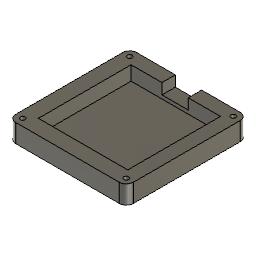
Abhay's+Macropad+Bottom (Autodesk Fusion 360 design; units mm, degrees)
part number: 2026-01-28-15-56-50-540
Autodesk Fusion 360 part; units mm, degrees
sketch "Sketch1" plane through (0, 0, 0) normal (0, 0, 1) x (1, 0, 0)
  line L0 (55, 35) -> (117.913, 35)
  line L1 (117.913, 35) -> (117.913, -30.294)
  line L2 (117.913, -30.294) -> (55, -30.294)
  line L3 (55, -30.294) -> (55, 35)
  line L4 (44.5, -40.794) -> (127.413, -40.794)
  line L5 (127.413, -40.794) -> (127.413, 44.5)
  line L6 (127.413, 44.5) -> (44.5, 44.5)
  line L7 (44.5, 44.5) -> (44.5, -40.794)
  circle A0 centre (49.5, -35.794) radius 1.7
  circle A1 centre (49.5, 39.5) radius 1.7
  circle A2 centre (122.413, 39.5) radius 1.7
  circle A3 centre (122.413, -35.794) radius 1.7
  circle A4 centre (49.5, -35.794) radius 3
  circle A5 centre (49.5, 39.5) radius 3
  circle A6 centre (122.413, 39.5) radius 3
  circle A7 centre (122.413, -35.794) radius 3
  dimension "d1" = 62.913
  dimension "d2" = 65.294
  dimension "d3" = 82.913
  dimension "d4" = 85.294
  dimension "d5" = 9.5
  dimension "d6" = 9.5
  dimension "d7" = 3.4
  dimension "d8" = 3.4
  dimension "d9" = 3.4
  dimension "d10" = 3.4
  dimension "d11" = 5
  dimension "d12" = 5
  dimension "d13" = 5
  dimension "d14" = 5
  dimension "d15" = 5
  dimension "d16" = 5
  dimension "d17" = 5
  dimension "d18" = 5
  dimension "d19" = 6
  dimension "d20" = 6
  dimension "d21" = 6
  dimension "d22" = 6
  constraint horizontal L0
  constraint vertical L1
  constraint horizontal L2
  constraint vertical L3
  constraint horizontal L4
  constraint vertical L5
  constraint horizontal L6
  constraint vertical L7
  constraint concentric A0 A4
  constraint concentric A1 A5
  constraint concentric A2 A6
  constraint concentric A3 A7
  measures "d1" distance of L0.start L0.end
  measures "d2" distance of L0.start L2.end
  measures "d3" distance of L4.start L4.end
  measures "d4" distance of L4.start L6.end
  measures "d5" distance of L0 L6
  measures "d6" distance of L1 L5
  measures "d7" diameter of A0
  measures "d8" diameter of A1
  measures "d9" diameter of A2
  measures "d10" diameter of A3
  measures "d11" distance of L4 A3.centre
  measures "d12" distance of L5 A3.centre
  measures "d13" distance of L6 A2.centre
  measures "d14" distance of L5 A2.centre
  measures "d15" distance of L6 A1.centre
  measures "d16" distance of L7 A1.centre
  measures "d17" distance of L4 A0.centre
  measures "d18" distance of L7 A0.centre
  measures "d19" diameter of A4
  measures "d20" diameter of A5
  measures "d21" diameter of A6
  measures "d22" diameter of A7
extrude "Extrude1" add sketch "Sketch1" along normal blind 9.9 from surface at 3.1 contours A4 | A5 | A6 | A7 makes body 1 at (123.2255, -32.9061, 9.7) makes body 2 at (123.2255, 42.3879, 9.7) makes body 3 at (46.5037, -35.9435, 9.7) makes body 4 at (46.5037, 39.3505, 9.7)
extrude "Extrude2" add sketch "Sketch1" along normal blind 13 contours L4 L5 L6 L7 bodies 1 2 3 4
extrude "Extrude3" add sketch "Sketch1" along normal blind 3 contours L0 L1 L2 L3 bodies 1
sketch "Sketch2" plane through (0, 0, 13) normal (0, 0, 1) x (-1, 0, 0)
  circle A0 centre (-122.413, 35.794) radius 1.7
  circle A1 centre (-49.5, -39.5) radius 1.7
  line L0 (-117.913, 30.294) -> (-55, 30.294)
  line L1 (-55, 30.294) -> (-55, -35)
  line L2 (-55, -35) -> (-117.913, -35)
  line L3 (-117.913, -35) -> (-117.913, 30.294)
  line L4 (-44.5, -44.5) -> (-44.5, 40.794)
  line L5 (-44.5, 40.794) -> (-127.413, 40.794)
  line L6 (-127.413, 40.794) -> (-127.413, -44.5)
  line L7 (-127.413, -44.5) -> (-44.5, -44.5)
  circle A2 centre (-122.413, -39.5) radius 1.7
  circle A3 centre (-49.5, 35.794) radius 1.7
  line L8 (-76.7065, -44.5) -> (-95.2065, -44.5)
  line L9 (-95.2065, -44.5) -> (-95.2065, -35)
  line L10 (-95.2065, -35) -> (-76.7065, -35)
  line L11 (-76.7065, -35) -> (-76.7065, -44.5)
  line L12 (-44.5, -44.5) -> (-44.5, 40.794)
  dimension "d30" = 18.5
  dimension "d31" = 32.2065
  constraint horizontal L8
  constraint vertical L9
  constraint horizontal L10
  constraint vertical L11
  constraint coincident L7 L8.start
  measures "d30" distance of L8.start L8.end
  measures "d31" distance of L11 L12
extrude "Extrude4" cut sketch "Sketch2" against normal blind 7.5 contours L2 L7 L8 L9 L10 L11 bodies 1
fillet "Fillet1" radius 5 4 edges at (44.5, 44.5, 6.5) (44.5, -40.794, 6.5) (127.413, 44.5, 6.5) (127.413, -40.794, 6.5) on bodies 1
sketch "Sketch3" plane through (0, 0, 13) normal (0, 0, 1) x (-1, 0, 0)
  circle A0 centre (-49.5, 35.794) radius 1.7
  circle A1 centre (-122.413, -39.5) radius 1.7
  arc A2 (-122.413, 40.794) -> (-127.413, 35.794) centre (-122.413, 35.794) ccw
  line L0 (-127.413, 35.794) -> (-127.413, -39.5)
  arc A3 (-127.413, -39.5) -> (-122.413, -44.5) centre (-122.413, -39.5) ccw
  line L1 (-122.413, -44.5) -> (-95.2065, -44.5)
  line L2 (-95.2065, -44.5) -> (-95.2065, -35)
  line L3 (-95.2065, -35) -> (-117.913, -35)
  line L4 (-117.913, -35) -> (-117.913, 30.294)
  line L5 (-117.913, 30.294) -> (-55, 30.294)
  line L6 (-55, 30.294) -> (-55, -35)
  line L7 (-55, -35) -> (-76.7065, -35)
  line L8 (-76.7065, -35) -> (-76.7065, -44.5)
  line L9 (-76.7065, -44.5) -> (-49.5, -44.5)
  arc A4 (-49.5, -44.5) -> (-44.5, -39.5) centre (-49.5, -39.5) ccw
  line L10 (-44.5, -39.5) -> (-44.5, 35.794)
  arc A5 (-44.5, 35.794) -> (-49.5, 40.794) centre (-49.5, 35.794) ccw
  line L11 (-49.5, 40.794) -> (-122.413, 40.794)
  circle A6 centre (-49.5, -39.5) radius 1.7
  circle A7 centre (-122.413, 35.794) radius 1.7
sketch "Sketch4" plane through (0, 0, 13) normal (0, 0, 1) x (-1, 0, 0)
